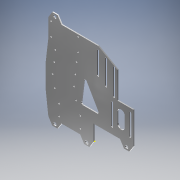
# Autodesk Inventor part: base_plate
Saved by Autodesk Inventor 2018 (Build 220112000, 112)
## iProperties
Created: 2018-04-04
Part Number: base_plate
Material: アルミニウム 6061
Document SubType Name: モデリング
Designer: NaMACHAN
Density: 2.7 g/cm^3
Appearance: アルミニウム - フラット
Sheet Metal Rule: Default
Mass: 92.2429 g
Surface Area: 369.048 cm^2
Volume: 34.164 cm^3
Author: NaMACHAN
Autodesk Inventor part; units mm, degrees
ref_plane "YZ Plane" through (0, 0, 0) normal (1, 0, 0) x (0, 1, 0)
ref_plane "XZ Plane" through (0, 0, 0) normal (0, 1, 0) x (-1, 0, 0)
ref_plane "XY Plane" through (0, 0, 0) normal (0, 0, 1) x (1, 0, 0)
sketch "スケッチ1" plane through (0, 0, 0) normal (0, 1, 0) x (-1, 0, 0)
  line L0 (85, 0) -> (90, 42)
  line L1 (90, 42) -> (90, 84)
  line L2 (90, 84) -> (85, 126)
  line L3 (-45, 90) -> (-45, 140)
  line L4 (0, 0) -> (0, 30)
  line L5 (-75, 90) -> (-45, 90)
  line L6 (77.5, 173) -> (67.5, 173)
  line L7 (60, 161) -> (67.5, 173)
  line L8 (85, 0) -> (77.5, -12)
  line L9 (77.5, -12) -> (67.5, -12)
  line L10 (67.5, -12) -> (60, 0)
  line L11 (60, 0) -> (25, 0)
  line L12 (25, 0) -> (17.5, -12)
  line L13 (17.5, -12) -> (7.5, -12)
  line L14 (7.5, -12) -> (0, 0)
  line L15 (0, 30) -> (-50, 30)
  line L16 (-50, 30) -> (-57.5, 18)
  line L17 (-57.5, 18) -> (-67.5, 18)
  line L18 (-67.5, 18) -> (-75, 30)
  line L19 (-75, 90) -> (-75, 30)
  line L20 (60, 161) -> (-8.6269, 161)
  line L21 (77.5, 173) -> (85, 161)
  line L22 (85, 161) -> (85, 126)
  line L23 (-8.6269, 161) -> (-19.0192, 155)
  line L24 (-19.0192, 155) -> (-32.0096, 162.5)
  line L25 (-32.0096, 162.5) -> (-40.6699, 157.5)
  line L26 (-40.6699, 157.5) -> (-40.6699, 142.5)
  line L27 (-40.6699, 142.5) -> (-45, 140)
  line L28 (-40.6699, 142.5) -> (-47.1651, 153.75) construction
  line L29 (-40.6699, 157.5) -> (-47.1651, 153.75) construction
  line L30 (-32.0096, 162.5) -> (-25.5144, 166.25) construction
  line L31 (-25.5144, 166.25) -> (-19.0192, 155) construction
  dimension "d219" = 30
  dimension "d224" = 10
  dimension "d227" = 7.5
  dimension "d233" = 10
  dimension "d234" = 10
  dimension "d235" = 7.5
  dimension "d236" = 7.5
  dimension "d238" = 7.5
  dimension "d240" = 10
  dimension "d241" = 7.5
  dimension "d242" = 12
  dimension "d276" = 7.5
  dimension "d277" = 60
  dimension "d278" = 5
  dimension "d282" = 42
  dimension "d283" = 42
  dimension "d284" = 42
  dimension "d285" = 7.5
  dimension "d286" = 12
  dimension "d287" = 7.5
  dimension "d288" = 90
  dimension "d290" = 30
  dimension "d302" = 35
  dimension "d303" = 130
  dimension "d346" = 50
  dimension "d347" = 12
  dimension "d349" = 150
  dimension "d350" = 10
  dimension "d352" = 30
  dimension "d353" = 7.5
  dimension "d354" = 7.5
  dimension "d355" = 5
  constraints: 64 end point, 5 horizontal alignment, 4 horizontal, 4 parallel, 4 perpendicular, 4 vertical, 2 collinear, 2 vertical alignment, 1 coincident, 1 point on line
  measures "d219" distance of L5.start L3.start
  measures "d224" distance of L6.start L6.end
  measures "d227" horizontal distance of L6.end L7.start
  measures "d233" distance of L8.end L9.end
  measures "d234" distance of L12.end L13.end
  measures "d235" horizontal distance of L0.start L8.end
  measures "d236" horizontal distance of point (0, 0) L13.end
  measures "d238" horizontal distance of L10.end L9.end
  measures "d240" distance of L16.end L17.end
  measures "d241" horizontal distance of L16.end L15.end
  measures "d242" distance from line of L18.end L17
  measures "d276" horizontal distance of L18.end L17.end
  measures "d277" distance of L5.start L18.end
  measures "d278" distance from line of L1 L2.end
  measures "d282" vertical distance of L2.end L1.end
  measures "d283" distance of L0.end L1.end
  measures "d284" vertical distance of L0.start L0.end
  measures "d285" horizontal distance of L11.end L12.end
  measures "d286" distance from line of L0.start L9
  measures "d287" horizontal distance of L2.end L6.start
  measures "d288" distance between parallel lines of L1 L4
  measures "d290" distance of L4.start L4.end
  measures "d302" distance of L21.end L2.end
  measures "d303" distance from line of L22 L3.end
  measures "d346" distance of L3.start L3.end
  measures "d347" distance from line of L21.end L6
  measures "d349" angle of L20 L23
  measures "d350" distance of L24.end L25.end
  measures "d352" angle of L26 L28
  measures "d353" distance of L25.end L28.end
  measures "d354" distance of L24.end L30.end
  measures "d355" distance of L26.end L3.end
extrude "押し出し1" add sketch "スケッチ1" along normal blind 2
fillet "フィレット1" radius 2 3 edges at (-85, 1, 126) (0, 1, 0) (-85, 1, 0)
sketch "スケッチ8" plane through (0, 2, 0) normal (0, 1, 0) x (1, 0, 0)
  point P0 (0, 0)
  point P1 (-65, -9.5)
  point P2 (-25, -9.5)
  point P3 (-25, -30.5)
  point P4 (-65, -30.5)
  point P5 (-73, -51.5)
  point P6 (-33, -51.5)
  point P7 (-77, -72.5)
  point P8 (-37, -72.5)
  point P9 (-34, -93.5)
  point P10 (-74, -93.5)
  point P11 (-72, -114.5)
  point P12 (-32, -114.5)
  dimension "d132" = 40
  dimension "d133" = 40
  dimension "d134" = 40
  dimension "d135" = 40
  dimension "d136" = 40
  dimension "d137" = 40
  dimension "d138" = 9.5
  dimension "d139" = 25
  dimension "d141" = 21
  dimension "d143" = 21
  dimension "d144" = 21
  dimension "d145" = 21
  dimension "d146" = 21
  dimension "d147" = 8
  dimension "d148" = 4
  dimension "d149" = 3
  dimension "d150" = 2
  constraints: 6 horizontal alignment, 1 vertical alignment
  measures "d132" distance of point (-25, -9.5) point (-65, -9.5)
  measures "d133" distance of point (-65, -30.5) point (-25, -30.5)
  measures "d134" distance of point (-73, -51.5) point (-33, -51.5)
  measures "d135" distance of point (-77, -72.5) point (-37, -72.5)
  measures "d136" distance of point (-34, -93.5) point (-74, -93.5)
  measures "d137" distance of point (-32, -114.5) point (-72, -114.5)
  measures "d138" vertical distance of point (0, 0) point (-25, -9.5)
  measures "d139" horizontal distance of point (0, 0) point (-25, -9.5)
  measures "d141" distance of point (-25, -30.5) point (-25, -9.5)
  measures "d143" vertical distance of point (-33, -51.5) point (-25, -30.5)
  measures "d144" vertical distance of point (-37, -72.5) point (-33, -51.5)
  measures "d145" vertical distance of point (-34, -93.5) point (-37, -72.5)
  measures "d146" vertical distance of point (-32, -114.5) point (-34, -93.5)
  measures "d147" horizontal distance of point (-25, -30.5) point (-33, -51.5)
  measures "d148" horizontal distance of point (-37, -72.5) point (-33, -51.5)
  measures "d149" horizontal distance of point (-34, -93.5) point (-37, -72.5)
  measures "d150" horizontal distance of point (-34, -93.5) point (-32, -114.5)
hole "穴6" at (-65, 2, 9.5) at (-25, 2, 9.5) at (-25, 2, 30.5) at (-65, 2, 30.5) at (-73, 2, 51.5) at (-33, 2, 51.5) at (-77, 2, 72.5) at (-37, 2, 72.5) at (-34, 2, 93.5) at (-74, 2, 93.5) at (-72, 2, 114.5) at (-32, 2, 114.5) direction (0, -1, 0) diameter 3 end through all
sketch "スケッチ11" plane through (0, 2, 0) normal (0, 1, 0) x (1, 0, 0)
  line L0 (25.6269, -93) -> (25.6269, -141)
  arc A0 (21.6269, -141) -> (25.6269, -141) centre (23.6269, -141) ccw
  line L1 (21.6269, -141) -> (21.6269, -93)
  arc A1 (25.6269, -93) -> (21.6269, -93) centre (23.6269, -93) ccw
  line L2 (-4.3731, -113) -> (-4.3731, -153)
  arc A2 (-8.3731, -153) -> (-4.3731, -153) centre (-6.3731, -153) ccw
  line L3 (-8.3731, -153) -> (-8.3731, -113)
  arc A3 (-4.3731, -113) -> (-8.3731, -113) centre (-6.3731, -113) ccw
  arc A4 (6.6269, -147) -> (10.6269, -147) centre (8.6269, -147) ccw
  line L4 (6.6269, -147) -> (6.6269, -103)
  arc A5 (10.6269, -103) -> (6.6269, -103) centre (8.6269, -103) ccw
  line L5 (10.6269, -103) -> (10.6269, -147)
  line L6 (-60, -161) -> (8.6269, -161) projected
  point P0 (0, 0)
  point P1 (50, -163)
  dimension "d194" = 2
  dimension "d198" = 2
  dimension "d295" = 2
  dimension "d298" = 2
  dimension "d308" = 8
  dimension "d309" = 15
  dimension "d311" = 15
  dimension "d314" = 40
  dimension "d315" = 10
  dimension "d316" = 10
  dimension "d319" = 6
  dimension "d320" = 6
  dimension "d348" = 15
  constraints: 12 end point, 12 point on circle, 9 tangent, 6 centre point, 3 parallel, 3 vertical, 2 horizontal alignment
  measures "d194" radius of A1
  measures "d198" radius of A2
  measures "d295" radius of A5
  measures "d298" radius of A4
  measures "d308" distance from line of L6 A2.centre
  measures "d309" horizontal distance of A2.centre A4.centre
  measures "d311" horizontal distance of A4.centre A0.centre
  measures "d314" distance of A2.centre A3.centre
  measures "d315" vertical distance of A3.centre A5.centre
  measures "d316" vertical distance of A1.centre A5.centre
  measures "d319" vertical distance of A2.centre A4.centre
  measures "d320" vertical distance of A0.centre A4.centre
  measures "d348" horizontal distance of L6.end A2.centre
extrude "押し出し3" cut sketch "スケッチ11" against normal blind 3
sketch "スケッチ12" plane through (0, 2, 0) normal (0, 1, 0) x (1, 0, 0)
  point P0 (0, 0)
sketch "スケッチ13" plane through (0, 2, 0) normal (0, 1, 0) x (1, 0, 0)
  line L0 (67, -82) -> (67, -43)
  arc A0 (71, -43) -> (67, -43) centre (69, -43) ccw
  line L1 (71, -43) -> (71, -82)
  arc A1 (67, -82) -> (71, -82) centre (69, -82) ccw
  line L2 (37, -82) -> (37, -43)
  arc A2 (37, -43) -> (33, -43) centre (35, -43) ccw
  line L3 (33, -43) -> (33, -82)
  arc A3 (33, -82) -> (37, -82) centre (35, -82) ccw
  line L4 (45, -90) -> (75, -90) projected
  line L5 (50, -30) -> (0, -30) projected
  line L6 (75, -90) -> (75, -30) projected
  point P0 (0, 0)
  dimension "d205" = 2
  dimension "d206" = 2
  dimension "d208" = 8
  dimension "d210" = 34
  dimension "d292" = 6
  dimension "d344" = 13
  constraints: 8 end point, 8 point on circle, 8 tangent, 4 centre point, 2 horizontal alignment, 2 parallel, 2 vertical
  measures "d205" radius of A3
  measures "d206" radius of A1
  measures "d208" distance from line of L4 A1.centre
  measures "d210" distance of A0.centre A2.centre
  measures "d292" distance from line of L6 A0.centre
  measures "d344" vertical distance of L6.end A0.centre
extrude "押し出し4" cut sketch "スケッチ13" against normal blind 10
sketch "スケッチ14" plane through (0, 0, 0) normal (0, -1, 0) x (1, 0, 0)
  line L0 (-67.5, 173) -> (-77.5, 173) projected
  line L1 (-77.5, -12) -> (-67.5, -12) projected
  line L2 (-17.5, -12) -> (-7.5, -12) projected
  line L3 (57.5, 18) -> (67.5, 18) projected
  line L4 (40.6699, 157.5) -> (32.0096, 162.5) projected
  line L5 (33.8397, 155.6699) -> (29.5096, 158.1699) construction
  line L6 (29.5096, 158.1699) -> (32.0096, 162.5) construction
  point P0 (0, 0)
  point P1 (-72.5, -7)
  point P2 (-12.5, -7)
  point P3 (-72.5, 168)
  point P4 (62.5, 23)
  point P5 (-72.5, 173)
  point P6 (-72.5, -12)
  point P7 (-12.5, -12)
  point P8 (62.5, 18)
  dimension "d245" = 5
  dimension "d246" = 5
  dimension "d247" = 5
  dimension "d248" = 5
  dimension "d356" = 5
  dimension "d357" = 5
  constraints: 4 end point, 4 midpoint, 4 vertical alignment, 2 perpendicular
  measures "d245" distance from line of point (-72.5, 168) L0
  measures "d246" distance from line of L1 point (-72.5, -7)
  measures "d247" distance of point (-12.5, -12) point (-12.5, -7)
  measures "d248" distance from line of L3 point (62.5, 23)
  measures "d356" distance from line of L4 L5.start
  measures "d357" distance of L5.start L5.end
hole "穴9" at (-72.5, 0, 168) at (-72.5, 0, -7) at (-12.5, 0, -7) at (62.5, 0, 23) at (33.8397, 0, 155.6699) direction (0, 1, 0) diameter 6 end through all
sketch "スケッチ16" plane through (0, 2, 0) normal (0, 1, 0) x (1, 0, 0)
  line L0 (-12.0233, -91.3731) -> (9.2654, -54.5)
  arc A0 (9.2654, -54.5) -> (6.6673, -50) centre (6.6673, -53) ccw
  line L1 (6.6673, -50) -> (-20, -50)
  arc A1 (-20, -50) -> (-22.5981, -54.5) centre (-20, -53) ccw
  line L2 (-22.5981, -54.5) -> (-17.9767, -91.3731)
  arc A2 (-17.9767, -91.3731) -> (-12.0233, -91.3731) centre (-15, -91) ccw
  line L3 (50, -30) -> (0, -30) projected
  line L4 (-60, -161) -> (8.6269, -161) projected
  line L5 (-85, -126.1186) -> (-85, -161) projected
  point P0 (0, 0)
  dimension "d264" = 20
  dimension "d266" = 20
  dimension "d267" = 3
  dimension "d268" = 3
  dimension "d269" = 3
  dimension "d270" = 120
  dimension "d271" = 120
  dimension "d317" = 70
  dimension "d318" = 70
  constraints: 6 end point, 6 point on circle, 4 tangent, 3 centre point, 1 horizontal, 1 horizontal alignment
  measures "d264" distance between parallel lines of L3 L1
  measures "d266" horizontal distance of A1.centre L3.end
  measures "d267" radius of A1
  measures "d268" radius of A0
  measures "d269" radius of A2
  measures "d317" distance from line of L4 A2.centre
  measures "d318" distance from line of L5 A2.centre
extrude "押し出し6" cut sketch "スケッチ16" against normal blind 10
sketch "スケッチ17" plane through (0, 2, 0) normal (0, 1, 0) x (1, 0, 0)
  point P0 (0, 0)
sketch "スケッチ18" plane through (0, 2, 0) normal (0, 1, 0) x (1, 0, 0)
  line L0 (45, -53) -> (45, -72)
  arc A0 (45, -72) -> (59, -72) centre (52, -72) ccw
  line L1 (59, -72) -> (59, -53)
  arc A1 (59, -53) -> (45, -53) centre (52, -53) ccw
  line L2 (37, -43) -> (37, -82) projected
  line L3 (67, -82) -> (67, -43) projected
  point P0 (0, 0)
  dimension "d321" = 30
  dimension "d322" = 15
  dimension "d323" = 10
  dimension "d324" = 10
  dimension "d325" = 7
  constraints: 4 end point, 4 point on circle, 4 tangent, 2 centre point, 1 parallel, 1 vertical
  measures "d321" distance between parallel lines of L2 L3
  measures "d322" distance from line of L3 A1.centre
  measures "d323" vertical distance of L3.start A0.centre
  measures "d324" vertical distance of L3.end A1.centre
  measures "d325" radius of A0
extrude "押し出し7" cut sketch "スケッチ18" against normal blind 10
sketch "スケッチ19" plane through (0, 2, 0) normal (0, 1, 0) x (1, 0, 0)
  line L0 (-60, -161) -> (8.6269, -161) projected
  line L1 (-85, -126.1186) -> (-85, -161) projected
  point P0 (-79.92, -131.79)
  point P1 (-29.12, -131.79)
  point P2 (-29.12, -157.19)
  point P3 (-79.92, -157.19)
  dimension "d333" = 50.8
  dimension "d334" = 25.4
  dimension "d335" = 3.81
  dimension "d336" = 5.08
  constraints: 2 horizontal alignment, 2 vertical alignment
  measures "d333" distance of point (-79.92, -157.19) point (-29.12, -157.19)
  measures "d334" distance of point (-79.92, -131.79) point (-79.92, -157.19)
  measures "d335" distance from line of L0 point (-79.92, -157.19)
  measures "d336" distance from line of L1 point (-79.92, -157.19)
hole "穴10" at (-79.92, 2, 157.19) at (-79.92, 2, 131.79) at (-29.12, 2, 131.79) at (-29.12, 2, 157.19) direction (0, -1, 0) diameter 3 end through all
